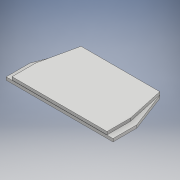
# Autodesk Inventor part: Game_VenusAwards
Saved by Autodesk Inventor 2018 (Build 220112000, 112)
## iProperties
Created: 2021-04-21
Part Number: Game_VenusAwards
Material: Generic
Document SubType Name: Modeling
Designer: Bradley
Density: 1 g/cm^3
Appearance: Default
Author: Bradley
Autodesk Inventor part; units mm, degrees
ref_plane "YZ Plane" through (0, 0, 0) normal (1, 0, 0) x (0, 1, 0)
ref_plane "XZ Plane" through (0, 0, 0) normal (0, 1, 0) x (-1, 0, 0)
ref_plane "XY Plane" through (0, 0, 0) normal (0, 0, 1) x (1, 0, 0)
sketch "Sketch1" plane through (0, 0, 0) normal (0, 0, 1) x (1, 0, 0)
  line L0 (-36, -28.5) -> (36, -28.5)
  line L1 (36, -28.5) -> (36, -12.5)
  line L2 (36, -12.5) -> (26.5, 12.5)
  line L3 (26.5, 12.5) -> (-26.5, 12.5)
  line L4 (-26.5, 12.5) -> (-36, -12.5)
  line L5 (-36, -12.5) -> (-36, -28.5)
  point P0 (0, 0)
  point P1 (0, -28.5)
  point P2 (-31.25, 0)
  dimension "d0" = 72
  dimension "d1" = 41
  dimension "d2" = 53
  dimension "d3" = 16
  constraints: 12 end point, 2 equal length, 2 midpoint, 2 parallel, 1 horizontal, 1 horizontal alignment, 1 perpendicular, 1 vertical alignment
  measures "d0" distance of L0.start L0.end
  measures "d1" distance between parallel lines of L0 L3
  measures "d2" distance of L2.end L3.end
  measures "d3" distance of L4.end L0.start
extrude "Extrusion1" add sketch "Sketch1" along normal blind 1.94
pattern_linear "Rectangular Pattern1" count 2 spacing 2.1 along (0, 0, 1) of "Extrusion1"
sketch "Sketch2" plane through (-36, -28.5, 4.04) normal (0, 0, 1) x (1, 0, 0)
  line L0 (0, 0) -> (72, 0) projected
  line L1 (72, 0) -> (72, 16) projected
  line L2 (72, 16) -> (62.5, 41) projected
  line L3 (62.5, 41) -> (9.5, 41) projected
  line L4 (9.5, 41) -> (0, 16) projected
  line L5 (0, 16) -> (0, 0) projected
  line L6 (62.5, 41) -> (9.5, 41) projected
  line L7 (9.5, 41) -> (4, 16)
  line L8 (4, 16) -> (4, 0)
  line L9 (62.5, 41) -> (68, 16)
  line L10 (68, 16) -> (68, 0)
  line L11 (0, 0) -> (72, 0) projected
  point P0 (36, 28.5)
  dimension "d9" = 64
  constraints: 8 end point, 3 equal length, 2 perpendicular, 2 point on line
  measures "d9" distance between parallel lines of L10 L8
extrude "Extrusion2" cut sketch "Sketch2" against normal up to next contours L5 L4 L7 L8 L0 | L10 L9 L2 L1 L0
body "Solid1"
